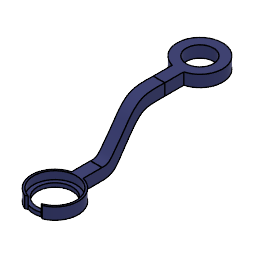
Armature 2 (Autodesk Fusion 360 design; units mm, degrees)
Autodesk Fusion 360 part; units mm, degrees
sketch "Counter holder" plane through (0, 0, 0) normal (0, 1, 0) x (1, 0, 0)
  line L0 (1.6795, -5.2373) -> (2.2579, -5.559)
  circle A0 centre (0, 0) radius 4.5
  line L1 (-1.6795, -5.2373) -> (-2.2579, -5.559)
  circle A1 centre (0, 0) radius 5.5
  arc A2 (2.2579, -5.559) -> (-1.5, 5.8095) centre (0, 0) ccw
  line L2 (0, 10.7) -> (-1.5, 10.7)
  line L3 (0, 10.7) -> (1.5, 10.7)
  arc A3 (-1.5, 5.8095) -> (-2.2579, -5.559) centre (0, 0) ccw
  line L4 (1.5, 10.7) -> (1.5, 5.8095)
  line L5 (-1.5, 10.7) -> (-1.5, 5.8095)
  point P0 (2.6505, 5.3709)
  dimension "d2" = 11
  dimension "d3" = 9
  dimension "d25" = 12
  dimension "d28" = 1.5
  dimension "d29" = 1.5
  constraint coincident L1.start A1
  constraint coincident A0.centre A1.centre
  constraint vertical L5
  constraint perpendicular L3 L4
  constraint concentric A2 A3
  constraint coincident A2 L4.end
  measures "d2" diameter of A1
  measures "d3" diameter of A0
  measures "d25" diameter of A2
  measures "d28" distance of L2.start L2.end
  measures "d29" distance of L2.start L3.end
ref_plane "WorkPlane1" through (0, 10.85, 0) normal (0, 1, 0) x (1, 0, 0)
sketch "Servo holder" plane through (0, 10.85, 0) normal (0, 1, 0) x (1, 0, 0)
  circle A0 centre (0, 37.482) radius 3.5
  line L0 (0.0036, 26.913) -> (-1.4964, 26.913)
  line L1 (-1.4964, 26.913) -> (0.0036, 26.913)
  line L2 (0.0036, 26.913) -> (1.5036, 26.913)
  line L3 (1.5036, 26.913) -> (1.5036, 31.8089)
  line L4 (-1.4964, 26.913) -> (-1.4964, 31.807)
  arc A1 (-1.4964, 31.807) -> (1.5036, 31.8089) centre (0, 37.482) ccw
  arc A2 (1.5036, 31.8089) -> (-1.4964, 31.807) centre (0, 37.482) ccw
  point P0 (2.4711, 32.1586)
  point P1 (-2.4665, 32.1565)
  dimension "d6" = 11.738
  dimension "d7" = 7
  dimension "d31" = 1.5
  dimension "d32" = 1.5
  constraint coincident P0 A1
  constraint coincident P1 A1
  constraint concentric A0 A1
  constraint perpendicular L2 L3
  constraint concentric A1 A2
  measures "d6" diameter of A1
  measures "d7" diameter of A0
  measures "d31" distance of L0.start L0.end
  measures "d32" distance of L0.start L2.end
extrude "Extrude4" add sketch "Counter holder" along normal blind 1 contours A1 makes body 1
extrude "Extrude5" add sketch "Counter holder" along normal blind 3 contours L0 L1 A1 A2 A3 bodies 1
extrude "Extrude6" add sketch "Counter holder" along normal blind 3 contours A2 L2 L3 L4 L5 bodies 1
extrude "Extrude7" add sketch "Servo holder" along normal blind 3 separate body contours A1 A2 makes body 2
extrude "Extrude8" add sketch "Servo holder" along normal blind 3 contours L0 L1 L2 L3 L4 A1 bodies 2
sketch "Connection" plane through (0, 0, 0) normal (1, 0, 0) x (0, 0, -1)
  line L0 (10.6742, 0.0115) -> (13.0212, 0.009) construction
  line L1 (13.0212, 0.009) -> (14.5207, 1.4657) construction
  line L2 (14.5207, 1.4657) -> (15.3617, 2.9367) construction
  line L3 (15.3617, 2.9367) -> (16.5492, 4.5723) construction
  line L4 (16.5492, 4.5723) -> (17.7004, 6.3241) construction
  line L5 (17.7004, 6.3241) -> (18.7215, 7.7387) construction
  line L6 (18.7215, 7.7387) -> (20.0559, 9.518) construction
  line L7 (20.0559, 9.518) -> (21.6526, 10.8269) construction
  line L8 (21.6526, 10.8269) -> (23.6966, 10.8532) construction
  line L9 (23.6966, 10.8532) -> (26.9817, 10.8544) construction
  spline S0 degree 5 poles (10.6742, 0.0115) (13.0212, 0.009) (14.5207, 1.4657) (15.3617, 2.9367) (16.5492, 4.5723) (17.7004, 6.3241) (18.7215, 7.7387) (20.0559, 9.518) (21.6526, 10.8269) (23.6966, 10.8532) (26.9817, 10.8544) knots 0 0 0 0 0 0 0.166667 0.333333 0.5 0.666667 0.833333 1 1 1 1 1 1
  spline S1 degree 5 poles (10.6774, 2.9747) (12.3316, 2.8904) (12.9969, 4.0027) (15.0793, 6.5355) (15.9956, 8.0056) (17.0271, 9.3169) (17.9968, 10.9661) (19.6323, 12.6073) (21.0727, 13.6625) (23.6453, 13.9834) (26.9849, 13.8452) knots 0 0 0 0 0 0 0.166667 0.333333 0.5 0.666667 0.833333 1 1 1 1 1 1
  line L10 (10.6774, 2.9747) -> (12.3316, 2.8904) construction
  line L11 (12.3316, 2.8904) -> (12.9969, 4.0027) construction
  line L12 (12.9969, 4.0027) -> (15.0793, 6.5355) construction
  line L13 (15.0793, 6.5355) -> (15.9956, 8.0056) construction
  line L14 (15.9956, 8.0056) -> (17.0271, 9.3169) construction
  line L15 (17.0271, 9.3169) -> (17.9968, 10.9661) construction
  line L16 (17.9968, 10.9661) -> (19.6323, 12.6073) construction
  line L17 (19.6323, 12.6073) -> (21.0727, 13.6625) construction
  line L18 (21.0727, 13.6625) -> (23.6453, 13.9834) construction
  line L19 (23.6453, 13.9834) -> (26.9849, 13.8452) construction
  line L20 (10.6774, 2.9747) -> (10.6742, 0.0115)
  line L21 (26.9849, 13.8452) -> (26.9817, 10.8544)
  constraint perpendicular L0 L20
  constraint parallel L20 L21
extrude "Extrude9" add sketch "Connection" along normal mid plane 3 bodies 1 2
named bodies: "Counter holder", "Servo holder"
